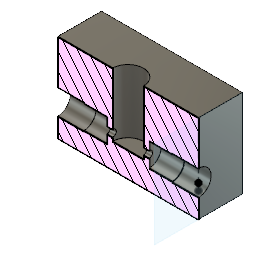
Brake Line Splitter v5 (Autodesk Fusion 360 design; units mm, degrees)
Autodesk Fusion 360 part; units mm, degrees
box "BoxPrimitive1" add length 25 width 40 height 25 placed x (0, 0, -1) y (-1, 0, 0) z (0, 1, 0) at (40, 0, 0)
hole "Hole1" at (20, 25, -12.5) direction (0, -1, 0) diameter 8.8 depth 18 tip angle 180
sketch "Sketch2" plane through (40, 0, 0) normal (1, 0, 0) x (0, 0, -1)
  line L0 (0, 25) -> (0, 0)
  line L1 (0, 0) -> (25, 0)
  line L2 (25, 0) -> (25, 25)
  line L3 (25, 25) -> (0, 25)
  line L4 (12.5, 25) -> (12.5, 7) construction
  point P0 (12.5, 9)
  dimension "d9" = 18
  dimension "d10" = 2
  constraint midpoint L3 L4.start
  constraint perpendicular L3 L4
  constraint coincident L4 P0
  measures "d9" distance of L4.start L4.end
  measures "d10" distance of L4.end P0
hole "Hole2" at (40, 9, -12.5) direction (-1, 0, 0) diameter 2 end through all
hole "Hole3" at (40, 9, -12.5) direction (-1, 0, 0) diameter 6.8 depth 14 tip angle 180
hole "Hole5" at (40, 9, -12.5) direction (-1, 0, 0) diameter 7.2 depth 7.5 tip angle 180
ref_plane "WorkPlane1" through (20, 12.5, -12.5) normal (-1, 0, 0) x (0, 1, 0)
mirror "Mirror1" about plane through (20, 12.5, -12.5) normal (-1, 0, 0) of "Hole3", "Hole5"
ref_plane "WorkPlane2" through (20, 12.5, -12.5) normal (0, 0, 1) x (0, 1, 0)
